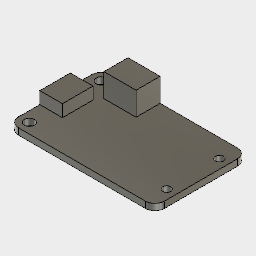
2465 Powerboost 1000C (Autodesk Fusion 360 design; units mm, degrees)
Autodesk Fusion 360 part; units mm, degrees
sketch "Sketch1" plane through (0, 0, 0) normal (0, 0, 1) x (1, 0, 0)
  line L0 (0, 0) -> (36.2, 0)
  line L1 (36.2, 0) -> (36.2, 22.86)
  line L2 (36.2, 22.86) -> (0, 22.86)
  line L3 (0, 22.86) -> (0, 0)
  circle A0 centre (2.54, 2.54) radius 1.25
  circle A1 centre (2.5529, 20.32) radius 1.25
  line L4 (14.67, 16.86) -> (6.67, 16.86)
  line L5 (6.67, 16.86) -> (6.67, 22.86)
  line L6 (6.67, 22.86) -> (14.67, 22.86)
  line L7 (14.67, 22.86) -> (14.67, 16.86)
  line L8 (14.67, 16.86) -> (6.67, 22.86) construction
  line L9 (6.67, 16.86) -> (14.67, 22.86) construction
  line L10 (5.65, 7.63) -> (0, 7.63)
  line L11 (0, 7.63) -> (0, 15.23)
  line L12 (0, 15.23) -> (5.65, 15.23)
  line L13 (5.65, 15.23) -> (5.65, 7.63)
  line L14 (5.65, 7.63) -> (0, 15.23) construction
  line L15 (0, 7.63) -> (5.65, 15.23) construction
  circle A2 centre (33.909, 18.3) radius 1
  line L16 (36.2, 11.43) -> (20, 11.43) construction
  circle A3 centre (33.909, 5.22) radius 1
  line L17 (36.2, 17.145) -> (20, 17.145) construction
  point P0 (10.67, 19.86)
  point P1 (2.825, 11.43)
  dimension "d1" = 36.2
  dimension "d2" = 22.86
  dimension "d3" = 2.5
  dimension "d4" = 2.54
  dimension "d5" = 2.54
  dimension "d6" = 2.5
  dimension "d9" = 8
  dimension "d10" = 6
  dimension "d11" = 10.67
  dimension "d13" = 5.65
  dimension "d14" = 7.6
  dimension "d16" = 2
  dimension "d45" = 11.43
  dimension "d46" = 17.78
  dimension "d47" = 2
  dimension "d49" = 13.08
  dimension "d50" = 5.715
  dimension "d51" = 33.909
  dimension "d52" = 33.909
  dimension "d53" = 5.22
  measures "d1" distance of L1.end L2.end
  measures "d2" distance of L0.start L2.end
  measures "d3" diameter of A0
  measures "d4" distance of L0 A0.centre
  measures "d5" distance of L3 A0.centre
  measures "d6" diameter of A1
  measures "d9" distance of L5.end L6.end
  measures "d10" distance of L4.end L5.end
  measures "d11" distance of L3 P0
  measures "d13" distance of L11.end L12.end
  measures "d14" distance of L10.end L11.end
  measures "d16" diameter of A2
  measures "d45" distance of L0 P1
  measures "d46" distance of A0.centre A1.centre
  measures "d47" diameter of A3
  measures "d49" distance of A2.centre A3.centre
  measures "d50" distance of L2 L17
  measures "d51" distance of L3 A3.centre
  measures "d52" distance of L3 A2.centre
  measures "d53" distance of L0 A3.centre
extrude "Extrude1" add sketch "Sketch1" against normal blind 1.6 makes body 1
fillet "Fillet1" radius 2.36 4 edges at (0, 0, -0.8) (0, 22.86, -0.8) (36.2, 22.86, -0.8) (36.2, 0, -0.8) on bodies 1
extrude "Extrude2" add sketch "Sketch1" along normal blind 3 separate body contours L3 L10 L11 L12 L13 makes body 2
extrude "Extrude3" add sketch "Sketch1" along normal blind 5.8 separate body contours L2 L4 L5 L6 L7 makes body 3
sketch "Sketch2" plane through (0, 0, -1.6) normal (0, 0, -1) x (1, 0, 0)
  arc A0 (36.2, -2.36) -> (33.84, 0) centre (33.84, -2.36) ccw construction
  line L0 (33.84, 0) -> (2.36, 0) construction
  arc A1 (2.36, 0) -> (0, -2.36) centre (2.36, -2.36) ccw construction
  line L1 (0, -2.36) -> (0, -20.5) construction
  arc A2 (0, -20.5) -> (2.36, -22.86) centre (2.36, -20.5) ccw construction
  line L2 (2.36, -22.86) -> (33.84, -22.86) construction
  arc A3 (33.84, -22.86) -> (36.2, -20.5) centre (33.84, -20.5) ccw construction
  line L3 (36.2, -20.5) -> (36.2, -2.36) construction
  circle A4 centre (2.5529, -20.32) radius 1.25
  circle A5 centre (33.909, -18.3) radius 1
  circle A6 centre (2.54, -2.54) radius 1.25
  circle A7 centre (2.54, -2.54) radius 2.5
  circle A8 centre (2.5529, -20.32) radius 2.5
  circle A9 centre (33.909, -5.22) radius 2.5
  circle A10 centre (33.909, -18.3) radius 2.5
  line L4 (17.78, 2) -> (17.78, -23.59) construction
  line L5 (16.2251, -15.6909) -> (19.2749, -6.3091) construction
  line L6 (30, -1) -> (5.5, -1)
  line L7 (5.5, -1) -> (5.5, -21)
  line L8 (5.5, -21) -> (30, -21)
  line L9 (30, -21) -> (30, -1)
  line L10 (30, -1) -> (5.5, -21) construction
  line L11 (5.5, -1) -> (30, -21) construction
  circle A11 centre (33.909, -5.22) radius 1
  line L12 (-2, -2.36) -> (-2, -20.5)
  arc A12 (-2, -20.5) -> (2.36, -24.86) centre (2.36, -20.5) ccw
  line L13 (2.36, -24.86) -> (33.84, -24.86)
  arc A13 (33.84, -24.86) -> (38.2, -20.5) centre (33.84, -20.5) ccw
  line L14 (38.2, -20.5) -> (38.2, -2.36)
  arc A14 (38.2, -2.36) -> (33.84, 2) centre (33.84, -2.36) ccw
  line L15 (33.84, 2) -> (2.36, 2)
  arc A15 (2.36, 2) -> (-2, -2.36) centre (2.36, -2.36) ccw
  point P0 (17.75, -11)
  dimension "d30" = 2
  dimension "d31" = 5
  dimension "d32" = 5
  dimension "d33" = 5
  dimension "d34" = 5
  measures "d31" diameter of A7
  measures "d32" diameter of A8
  measures "d33" diameter of A9
  measures "d34" diameter of A10
extrude "Extrude8" add sketch "Sketch2" along normal blind 3 separate body contours A4 | A5 | A6 | A7 | A8 | A9 | A10 | A11 makes body 4 at (36.3966, 18.5489, -2.6) makes body 5 at (5.0276, 2.7889, -2.6) makes body 6 at (5.0497, 20.4446, -3.6) makes body 7 at (36.3966, 5.4689, -2.6)
extrude "Extrude9" add sketch "Sketch2" along normal blind 4 and the other way blind -3 contours A4 | A5 | A6 | A7 | A8 | A9 | A10 | A11 | L12 A12 L13 A13 L14 A14 L15 A15 bodies 5 6 7 4
extrude "Extrude10" add sketch "Sketch2" against normal blind 2 contours A4 | A5 | A6 | A11 bodies 5
hidden bodies 5
